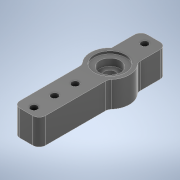
# Autodesk Inventor part: bottomsupport
Saved by Autodesk Inventor 2022 (Build 260153000, 153)
## iProperties
Created: 2022-03-10
Part Number: bottomsupport
Material: Genérico
Document SubType Name: Modeling
Designer: JK
Density: 1 g/cm^3
Appearance: Suave - Negro
Author: JK
Autodesk Inventor part; units mm, degrees
ref_plane "YZ Plane" through (0, 0, 0) normal (1, 0, 0) x (0, 1, 0)
ref_plane "XZ Plane" through (0, 0, 0) normal (0, 1, 0) x (-1, 0, 0)
ref_plane "XY Plane" through (0, 0, 0) normal (0, 0, 1) x (1, 0, 0)
sketch "Boceto1" plane through (0, 0, 0) normal (0, 1, 0) x (-1, 0, 0)
  line L0 (-10, 44.5408) -> (10, 44.5408)
  line L1 (10, 44.5408) -> (10, -27.9592)
  line L2 (10, -27.9592) -> (-10, -27.9592)
  line L3 (-10, -27.9592) -> (-10, 44.5408)
  line L4 (-10, 44.5408) -> (10, -27.9592) construction
  line L5 (10, 44.5408) -> (-10, -27.9592) construction
  circle A0 centre (0, -20.4592) radius 4.4
  point P0 (0, 8.2908)
  dimension "d1" = 20
  dimension "d2" = 8.8
  dimension "d3" = 7.5
  dimension "d26" = 65
  constraints: 12 end point, 2 midpoint, 2 parallel, 1 centre point, 1 horizontal, 1 perpendicular
  measures "d1" distance between parallel lines of L1 L3
  measures "d2" diameter of A0
  measures "d3" distance from line of L2 A0.centre
  measures "d26" distance from line of L0 A0.centre
extrude "Extrusión1" add sketch "Boceto1" along normal blind 20
sketch "Boceto2" plane through (0, 20, 0) normal (0, 1, 0) x (1, 0, 0)
  circle A0 centre (0, 20.4592) radius 4.4 projected
  circle A1 centre (0, 20.4592) radius 12.125
  point P0 (0, 0)
  dimension "d6" = 24.25
  constraints: 1 centre point, 1 coincident
  measures "d6" diameter of A1
extrude "Extrusión2" cut sketch "Boceto2" against normal blind 2.5
sketch "Boceto3" plane through (0, 20, 0) normal (0, 1, 0) x (1, 0, 0)
  circle A0 centre (0, 20.4592) radius 4.4 projected
  circle A1 centre (0, 20.4592) radius 12.125
  circle A2 centre (0, 20.4592) radius 15.125
  line L0 (10, 27.316) -> (10, 13.6024) projected
  arc A3 (10, 27.316) -> (9.5271, 27.9592) centre (0, 20.4592) ccw projected
  line L1 (-9.5271, 27.9592) -> (9.5271, 27.9592) projected
  arc A4 (-9.5271, 27.9592) -> (-10, 27.316) centre (0, 20.4592) ccw projected
  line L2 (-10, 13.6024) -> (-10, 27.316) projected
  arc A5 (-10, 13.6024) -> (10, 13.6024) centre (0, 20.4592) ccw projected
  circle A6 centre (0, 20.4592) radius 4.4 projected
  point P0 (0, 0)
  point P1 (-10, 27.316)
  point P2 (10, 27.316)
  point P3 (9.5271, 27.9592)
  dimension "d9" = 3
  constraints: 2 centre point, 2 coincident
  measures "d9" radial gap between concentric circles of A2 A1
extrude "Extrusión3" add sketch "Boceto3" against normal up to surface (20 mm away) contours A1 L0 | L1 A1 | A1 L2 | A2
sketch "Boceto4" plane through (0, 20, 0) normal (0, 1, 0) x (1, 0, 0)
  circle A0 centre (0, 20.4592) radius 4.4 projected
  circle A1 centre (0, 20.4592) radius 12.15
  point P0 (0, 0)
  dimension "d14" = 24.3
  constraints: 1 centre point, 1 coincident
  measures "d14" diameter of A1
extrude "Extrusión4" cut sketch "Boceto4" against normal blind 2 contours A0 | A1
sketch "Boceto5" plane through (0, 17.5, 0) normal (0, 1, 0) x (1, 0, 0)
  line L0 (10, 27.316) -> (10, 13.6024) projected
  arc A0 (10, 27.316) -> (9.5271, 27.9592) centre (0, 20.4592) ccw projected
  line L1 (-9.5271, 27.9592) -> (9.5271, 27.9592) projected
  arc A1 (-9.5271, 27.9592) -> (-10, 27.316) centre (0, 20.4592) ccw projected
  line L2 (-10, 13.6024) -> (-10, 27.316) projected
  arc A2 (-10, 13.6024) -> (10, 13.6024) centre (0, 20.4592) ccw projected
  circle A3 centre (0, 20.4592) radius 4.4 projected
  point P0 (0, 0)
extrude "Extrusión5" add sketch "Boceto5" along normal up to surface (0.5 mm away)
sketch "Boceto6" plane through (0, 0, 0) normal (0, -1, 0) x (1, 0, 0)
  circle A0 centre (0, 38.5408) radius 2.7
  circle A1 centre (0, 22.5408) radius 2.7
  line L0 (-10, 44.5408) -> (10, 44.5408) projected
  circle A2 centre (0, 6.5408) radius 2.7
  point P0 (0, 0)
  dimension "d20" = 16
  dimension "d21" = 5.4
  dimension "d30" = 6
  dimension "d35" = 16
  constraints: 3 centre point, 2 equal radius
  measures "d20" distance of A1.centre A0.centre
  measures "d21" diameter of A0
  measures "d30" distance from line of L0 A0.centre
  measures "d35" distance of A1.centre A2.centre
extrude "Extrusión6" cut sketch "Boceto6" against normal through all
sketch "Boceto8" plane through (0, 18, -20.4592) normal (0, 1, 0) x (1, 0, 0)
  circle A0 centre (0, 0) radius 4.4 projected
  circle A1 centre (0, 0) radius 8.125
  point P0 (0, -20.4592)
  dimension "d31" = 16.25
  constraints: 1 centre point, 1 coincident
  measures "d31" diameter of A1
extrude "Extrusión8" cut sketch "Boceto8" against normal blind 5.5 contours A0 | A1
fillet "Empalme4" radius 5 4 edges at (10, 10, 44.5408) (-10, 10, 44.5408) (10, 10, -9.1117) (-10, 10, -9.1117)
sketch "Boceto9" plane through (0, 20, 0) normal (0, 1, 0) x (1, 0, 0)
  arc A0 (11.2733, 10.3756) -> (-11.2733, 10.3756) centre (0, 20.4592) ccw projected
  line L0 (-10, 31.8067) -> (10, 31.8067)
  line L1 (10, 31.8067) -> (10, 54.4592)
  line L2 (10, 54.4592) -> (-10, 54.4592)
  line L3 (-10, 54.4592) -> (-10, 31.8067)
  line L4 (-10, 7.0422) -> (-10, -39.5408) projected
  line L5 (10, -39.5408) -> (10, 7.0422) projected
  circle A1 centre (0, 20.4592) radius 21
  circle A2 centre (0, 47.4592) radius 2.7
  point P0 (0, 0)
  dimension "d36" = 42
  dimension "d37" = 34
  dimension "d38" = 5.4
  dimension "d39" = 7
  constraints: 8 end point, 2 centre point, 2 collinear, 2 parallel, 1 coincident, 1 horizontal, 1 perpendicular, 1 point on circle
  measures "d36" diameter of A1
  measures "d37" distance from line of L2 A0.centre
  measures "d38" diameter of A2
  measures "d39" distance from line of L2 A2.centre
extrude "Extrusión9" add sketch "Boceto9" against normal up to surface (20 mm away) contours A0 L3 A1 L1 | A1 L3 L2 L1
fillet "Empalme5" radius 5 3 edges at (10, 10, -31.8067) (10, 10, -54.4592) (-10, 10, -54.4592)
sketch "Boceto10" plane through (0, 0, 0) normal (0, -1, 0) x (1, 0, 0)
  circle A0 centre (0, -47.4592) radius 2.7 projected
  circle A1 centre (0, -47.4592) radius 4
  circle A2 centre (0, 6.5408) radius 2.7 projected
  circle A3 centre (0, 6.5408) radius 4
  line L0 (-4.6188, -47.4592) -> (-2.3094, -43.4592)
  line L1 (-2.3094, -43.4592) -> (2.3094, -43.4592)
  line L2 (2.3094, -43.4592) -> (4.6188, -47.4592)
  line L3 (4.6188, -47.4592) -> (2.3094, -51.4592)
  line L4 (2.3094, -51.4592) -> (-2.3094, -51.4592)
  line L5 (-2.3094, -51.4592) -> (-4.6188, -47.4592)
  line L6 (-4.6188, 6.5408) -> (-2.3094, 10.5408)
  line L7 (-2.3094, 10.5408) -> (2.3094, 10.5408)
  line L8 (2.3094, 10.5408) -> (4.6188, 6.5408)
  line L9 (4.6188, 6.5408) -> (2.3094, 2.5408)
  line L10 (2.3094, 2.5408) -> (-2.3094, 2.5408)
  line L11 (-2.3094, 2.5408) -> (-4.6188, 6.5408)
  point P0 (0, 0)
  dimension "d43" = 8
  constraints: 24 end point, 4 coincident, 2 centre point, 2 horizontal, 2 tangent, 1 equal radius, 26 other
  measures "d43" diameter of A1
extrude "Extrusión10" cut sketch "Boceto10" against normal blind 4.2 contours A0 | A1 | A1 L2 L3 | A1 L1 L2 | L3 L4 A1 | A1 L0 L1 | L4 L5 A1 | A1 L5 L0 | A2 | A3 | A3 L8 L9 | A3 L7 L8 | L9 L10 A3 | A3 L6 L7 | L10 L11 A3 | A3 L11 L6
sketch "Boceto7" plane through (0, 0, 0) normal (0, -1, 0) x (1, 0, 0)
  circle A0 centre (0, -20.4592) radius 2.65 projected
  circle A1 centre (0, -20.4592) radius 4.05
  line L0 (0, -25.1357) -> (-4.05, -22.7975)
  line L1 (-4.05, -22.7975) -> (-4.05, -18.1209)
  line L2 (-4.05, -18.1209) -> (0, -15.7826)
  line L3 (0, -15.7826) -> (4.05, -18.1209)
  line L4 (4.05, -18.1209) -> (4.05, -22.7975)
  line L5 (4.05, -22.7975) -> (0, -25.1357)
  point P0 (0, 0)
  dimension "d27" = 8.1
  constraints: 12 end point, 2 coincident, 1 centre point, 1 tangent, 1 vertical, 13 other
  measures "d27" diameter of A1
